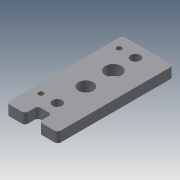
# Autodesk Inventor part: HbBatteryPcb01
Saved by Autodesk Inventor 2015 SP1 (Build 190203100, 203)
## iProperties
Created: 2015-03-05
Part Number: HbBatteryPcb01
Material: 一般
Document SubType Name: Modeling
Designer: Yamaura
Density: 1 g/cm^3
Appearance: 既定
Author: Yamaura
Autodesk Inventor part; units mm, degrees
ref_plane "YZ Plane" through (0, 0, 0) normal (1, 0, 0) x (0, 1, 0)
ref_plane "XZ Plane" through (0, 0, 0) normal (0, 1, 0) x (-1, 0, 0)
ref_plane "XY Plane" through (0, 0, 0) normal (0, 0, 1) x (1, 0, 0)
sketch "スケッチ1" plane through (0, 0, 0) normal (0, 0, 1) x (1, 0, 0)
  line L0 (4, 15.1) -> (12, 15.1)
  line L1 (12, 15.1) -> (12, -3)
  line L2 (4, -3) -> (4, 15.1)
  circle A0 centre (8, 9.7) radius 1.25 projected
  circle A1 centre (50, 5.4) radius 1.15 projected
  circle A2 centre (8, -5.4) radius 1.15 projected
  circle A3 centre (50, -5.4) radius 1.15 projected
  circle A4 centre (8, 5.4) radius 1.15 projected
  line L3 (-1, 21.7) -> (66, 21.7) projected
  line L4 (-2, 20.7) -> (-2, -20.7) projected
  line L5 (66, -21.7) -> (-1, -21.7) projected
  circle A5 centre (8, 13.15) radius 0.75
  circle A6 centre (8, 0.95) radius 0.75
  line L6 (6.8, 15.1) -> (9.4, 15.1)
  line L7 (9.1, -3) -> (9.1, -1)
  line L8 (9.1, -1) -> (6.9, -1)
  line L9 (6.9, -1) -> (6.9, -3)
  circle A7 centre (8, -5.4) radius 2
  line L10 (12, -3) -> (9.1, -3)
  line L11 (6.9, -3) -> (4, -3)
  line L12 (49.4, 10.95) -> (50.6, 10.95) projected
  arc A8 (51.5, 10.05) -> (50.6, 10.95) centre (50.6, 10.05) ccw projected
  line L13 (50.6, 8.45) -> (49.4, 8.45) projected
  arc A9 (48.5, 9.35) -> (49.4, 8.45) centre (49.4, 9.35) ccw projected
  arc A10 (66, -21.7) -> (67, -20.7) centre (66, -20.7) ccw projected
  arc A11 (67, 20.7) -> (66, 21.7) centre (66, 20.7) ccw projected
  arc A12 (-1, 21.7) -> (-2, 20.7) centre (-1, 20.7) ccw projected
  arc A13 (-2, -20.7) -> (-1, -21.7) centre (-1, -20.7) ccw projected
  line L14 (9.5, -0.55) -> (3.96, -0.55) projected
  line L15 (3.96, -0.55) -> (3.96, 2.45) projected
  line L16 (3.96, 2.45) -> (9.5, 2.45) projected
  line L17 (9.5, 2.45) -> (9.5, -0.55) projected
  line L18 (9.5, 11.65) -> (3.96, 11.65) projected
  line L19 (3.96, 11.65) -> (3.96, 14.65) projected
  line L20 (3.96, 14.65) -> (9.5, 14.65) projected
  line L21 (9.5, 14.65) -> (9.5, 11.65) projected
  line L22 (54, 9) -> (67, 9) projected
  line L23 (67, 20.7) -> (67, 9) projected
  line L24 (67, -7.5) -> (67, -20.7) projected
  line L25 (67, -7.5) -> (54, -7.5) projected
  line L26 (54, -7.5) -> (54, 9) projected
  line L27 (51.5, 10.05) -> (51.5, 9.35) projected
  arc A14 (50.6, 8.45) -> (51.5, 9.35) centre (50.6, 9.35) ccw projected
  line L28 (48.5, 9.35) -> (48.5, 10.05) projected
  arc A15 (49.4, 10.95) -> (48.5, 10.05) centre (49.4, 10.05) ccw projected
  point P0 (0, 0)
  point P1 (8, -2.2)
  dimension "d6" = 8
  dimension "d7" = 1.5
  dimension "d8" = 1.5
  dimension "d22" = 4
  dimension "d24" = 1.2
  dimension "d25" = 11.9
  dimension "d27" = 3
  dimension "d32" = 1.1
  dimension "d33" = 1.1
  dimension "d35" = 4.3
  dimension "d36" = 3.45
  dimension "d37" = 8.75
  dimension "d38" = 4.45
  constraints: 18 end point, 4 parallel, 3 centre point, 2 horizontal, 1 coincident, 1 perpendicular, 1 point on line
  measures "d6" distance of L0.start L0.end
  measures "d7" diameter of A5
  measures "d8" diameter of A6
  measures "d22" diameter of A7
  measures "d24" distance from line of L8 point (8, -2.2)
  measures "d25" distance of A0.centre point (8, -2.2)
  measures "d27" distance of L16.end L14.start
  measures "d32" distance from line of L9 point (8, -2.2)
  measures "d33" distance from line of L7 point (8, -2.2)
  measures "d35" distance of A4.centre A0.centre
  measures "d36" distance of A5.centre A0.centre
  measures "d37" distance of A6.centre A0.centre
  measures "d38" distance of A6.centre A4.centre
extrude "押し出し1" add sketch "スケッチ1" along normal blind 1.6 contours L0 L1 L10 L7 L8 L9 L11 L2 L14 L17 L16 L18 L21 L20 | L20 L21 L18 L2 | L16 L17 L14 L2
sketch "スケッチ2" plane through (0, 0, 1.6) normal (0, 0, 1) x (1, 0, 0)
  circle A0 centre (8, 13.15) radius 0.75 projected
  circle A1 centre (8, 0.95) radius 0.75 projected
  circle A2 centre (8, 9.7) radius 1.25 projected
  circle A3 centre (8, 5.4) radius 1.15 projected
  line L0 (12, 15.1) -> (4, 15.1) projected
  line L1 (4, 15.1) -> (4, -3) projected
  line L2 (9.1, -3) -> (12, -3) projected
  line L3 (12, -3) -> (12, 15.1) projected
  circle A4 centre (5.46, 13.15) radius 0.4
  circle A5 centre (5.46, 0.95) radius 0.4
  line L4 (4, -3) -> (6.9, -3) projected
  line L5 (6.9, -3) -> (6.9, -1) projected
  line L6 (6.9, -1) -> (9.1, -1) projected
  line L7 (9.1, -1) -> (9.1, -3) projected
  point P0 (0, 0)
  dimension "d11" = 0.8
  dimension "d12" = 0.8
  dimension "d13" = 2.54
  dimension "d14" = 2.54
  constraints: 2 centre point, 2 horizontal alignment
  measures "d11" diameter of A4
  measures "d12" diameter of A5
  measures "d13" distance of A4.centre A0.centre
  measures "d14" distance of A1.centre A5.centre
extrude "押し出し2" cut sketch "スケッチ2" against normal through all contours A4 | A5
fillet "フィレット1" radius 0.5 8 edges at (4, 15.1, 0.8) (4, -3, 0.8) (6.9, -3, 0.8) (6.9, -1, 0.8) (9.1, -1, 0.8) (9.1, -3, 0.8) (12, -3, 0.8) (12, 15.1, 0.8)
